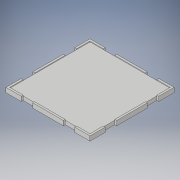
# Autodesk Inventor part: BT002_trajan20_21
Saved by Autodesk Inventor 2022.2 (Build 262287000, 287)
## iProperties
Company: HTBLA Kaindorf
RuleStatus: InUse
Created: 2022-08-01
Part Number: BT002_trajan20_21
Project: Zeichenmaschine_v2
Material: Generisch
Description: papierplatte
Document SubType Name: Modeling
Designer: trajan20
Density: 1 g/cm^3
Appearance: Vorgabe
Mass: 477.864 g
Surface Area: 1071.15 cm^2
Volume: 477.864 cm^3
AfterDocNew0: iProperties-Editor_aufrufen
Author: jan
Keywords: 2021
Autodesk Inventor part; units mm, degrees
ref_plane "YZ Plane" through (0, 0, 0) normal (1, 0, 0) x (0, 1, 0)
ref_plane "XZ Plane" through (0, 0, 0) normal (0, 1, 0) x (-1, 0, 0)
sketch "Skizze3" plane through (0, 0, 0) normal (0, 0, 1) x (1, 0, 0)
  line L0 (0, 0) -> (210, 0)
  line L1 (210, 0) -> (210, 210)
  line L2 (210, 210) -> (0, 210)
  line L3 (0, 210) -> (0, 0)
  line L4 (-5, 215) -> (215, 215)
  line L5 (215, 215) -> (215, -5)
  line L6 (215, -5) -> (-5, -5)
  line L7 (-5, -5) -> (-5, 215)
  line L8 (-5, 105) -> (215, 105)
  line L9 (105, 215) -> (105, -5)
  line L10 (-5, 65) -> (0, 65)
  line L11 (-5, 35) -> (0, 35)
  line L12 (35, -5) -> (35, 0)
  line L13 (65, -5) -> (65, 0)
  point P0 (210, 105)
  point P1 (105, 0)
  point P2 (105, 105)
  point P3 (0, 105)
  point P4 (122.5, 105)
  point P5 (105, 105)
  dimension "d4" = 210
  dimension "d5" = 210
  dimension "d6" = 220
  dimension "d7" = 220
  dimension "d8" = 5
  dimension "d9" = 5
  dimension "d12" = 30
  dimension "d13" = 40
  dimension "d14" = 30
  dimension "d15" = 40
  dimension "d27" = 17.5
  constraints: 28 end point, 9 point on line, 6 midpoint, 6 perpendicular, 4 parallel, 2 horizontal
  measures "d4" distance from line of point (210, 105) L3
  measures "d5" distance between parallel lines of L2 L0
  measures "d6" distance between parallel lines of L7 L5
  measures "d7" distance between parallel lines of L4 L6
  measures "d8" distance between parallel lines of L0 L6
  measures "d9" distance between parallel lines of L3 L7
  measures "d12" distance between parallel lines of L10 L11
  measures "d13" distance between parallel lines of L8 L10
  measures "d14" distance between parallel lines of L13 L12
  measures "d15" distance between parallel lines of L7 L12
  measures "d27" distance from line of L9 point (122.5, 105)
extrude "Extrusion3" add sketch "Skizze3" along normal blind 10 contours L3 L8 L9 L0
extrude "Extrusion4" add sketch "Skizze3" along normal blind 12 contours L0 L12 L6 L7 L11 L3 | L0 L9 L6 L13 | L10 L7 L8 L3
mirror "Spiegeln2" about plane through (105, 0, 0) normal (1, 0, 0) of "Extrusion3", "Extrusion4"
mirror "Spiegeln3" about plane through (105, 105, 0) normal (0, 1, 0) of "Extrusion3", "Extrusion4", "Spiegeln2"
hole "Bohrung1" at (122.5, 105, 0) direction (0, 0, 1) diameter 2.459 depth 8.8 tip angle 118 thread size "M3x0.5" class "6H" standard "ISO Metric profile"
ref_plane "Arbeitsebene1" through (105, 215, 0) normal (1, 0, 0) x (0, 1, 0)
hole "Bohrung2" at (105, 105, 0) direction (0, 0, 1) diameter 5 depth 4
pattern_circular "Runde Anordnung1" count 6 over 360 about axis through (105, 105, 2) along (0, 0, 1) of "Bohrung1"
equation "\"d7\" = d6"
equation "\"d14\" = d12"
equation "\"d15\" = d13"
